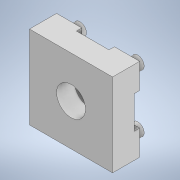
# Autodesk Inventor part: AS5600 Testteil
Saved by Autodesk Inventor 2021 (Build 250183000, 183)
## iProperties
Created: 2024-03-30
Part Number: AS5600 Testteil
Material: Generic
Document SubType Name: Modeling
Designer: Lukas
Density: 1 g/cm^3
Appearance: Default
Author: Lukas
Autodesk Inventor part; units mm, degrees
ref_plane "YZ Plane" through (0, 0, 0) normal (1, 0, 0) x (0, 1, 0)
ref_plane "XZ Plane" through (0, 0, 0) normal (0, 1, 0) x (-1, 0, 0)
ref_plane "XY Plane" through (0, 0, 0) normal (0, 0, 1) x (1, 0, 0)
sketch "Sketch1" plane through (0, 0, 0) normal (0, 0, 1) x (1, 0, 0)
  line L0 (11.5, -11.5) -> (-11.5, -11.5)
  line L1 (-11.5, -11.5) -> (-11.5, 11.5)
  line L2 (-11.5, 11.5) -> (11.5, 11.5)
  line L3 (11.5, 11.5) -> (11.5, -11.5)
  point P0 (0, 0)
  point P1 (0, 11.5)
  point P2 (-11.5, 0)
  dimension "d0" = 23
  constraints: 8 end point, 2 midpoint, 2 parallel, 2 perpendicular, 1 horizontal, 1 horizontal alignment, 1 vertical alignment
  measures "d0" distance of L1.end L2.end
extrude "Extrusion1" add sketch "Sketch1" along normal blind 6
sketch "Sketch2" plane through (0, 0, 6) normal (0, 0, 1) x (1, 0, 0)
  circle A0 centre (0, 0) radius 4
  dimension "d3" = 8
  constraints: 1 centre point, 1 coincident
  measures "d3" diameter of A0
extrude "Extrusion2" cut sketch "Sketch2" against normal blind 5
sketch "Sketch3" plane through (0, 0, 0) normal (0, 0, -1) x (-1, 0, 0)
  line L0 (11.5, 11.5) -> (11.5, -11.5) projected
  line L1 (11.5, -11.5) -> (4.5, -11.5)
  line L2 (4.5, -11.5) -> (4.5, -4.5)
  line L3 (4.5, -4.5) -> (11.5, -4.5)
  line L4 (11.5, -4.5) -> (11.5, -11.5)
  circle A0 centre (8, -8) radius 1.75
  point P0 (0, 0)
  dimension "d6" = 3.5
  dimension "d7" = 7
  dimension "d8" = 8
  dimension "d9" = 8
  constraints: 8 end point, 2 parallel, 2 perpendicular, 1 centre point, 1 horizontal
  measures "d6" diameter of A0
  measures "d7" distance of L1.end L2.end
  measures "d8" horizontal distance of point (0, 0) A0.centre
  measures "d9" horizontal distance of point (0, 0) A0.centre
extrude "Extrusion3" add sketch "Sketch3" along normal blind 1.5
extrude "Extrusion4" add sketch "Sketch3" along normal blind 4.5 contours A0
pattern_circular "Circular Pattern1" count 4 over 360 about axis through (0, 0, -10) along (0, 0, 1) of "Extrusion3", "Extrusion4"
equation "\"d9\" = d8"
body "Solid1"
